# Autodesk Inventor part: S2_PBTH
Saved by Autodesk Inventor 2016 SP1 (Build 200210100, 210)
## iProperties
Created: 2015-11-24
Part Number: S2_PBTH
Material: Generic
Document SubType Name: Modeling
Designer: PhillipD
Density: 1 g/cm^3
Appearance: PBTH, S2_PBTH
Author: PhillipD
Autodesk Inventor part; units mm, degrees
ref_plane "YZ Plane" through (0, 0, 0) normal (1, 0, 0) x (0, 1, 0)
ref_plane "XZ Plane" through (0, 0, 0) normal (0, 1, 0) x (-1, 0, 0)
ref_plane "XY Plane" through (0, 0, 0) normal (0, 0, 1) x (1, 0, 0)
sketch "PBTH, S2_PBTH_140" plane through (0, 0, 0) normal (0, 0, 1) x (1, 0, 0)
  line L0 (-0.548, 3.038) -> (5.6242, 3.038)
  line L1 (5.6242, 3.038) -> (5.6242, -3.058)
  line L2 (5.6242, -3.058) -> (-0.548, -3.058)
  line L3 (-0.548, -3.058) -> (-0.548, 3.038)
  constraints: 8 end point
extrude "Extrusion1" add sketch "PBTH, S2_PBTH_140" along normal blind 1
body "Solid1"
